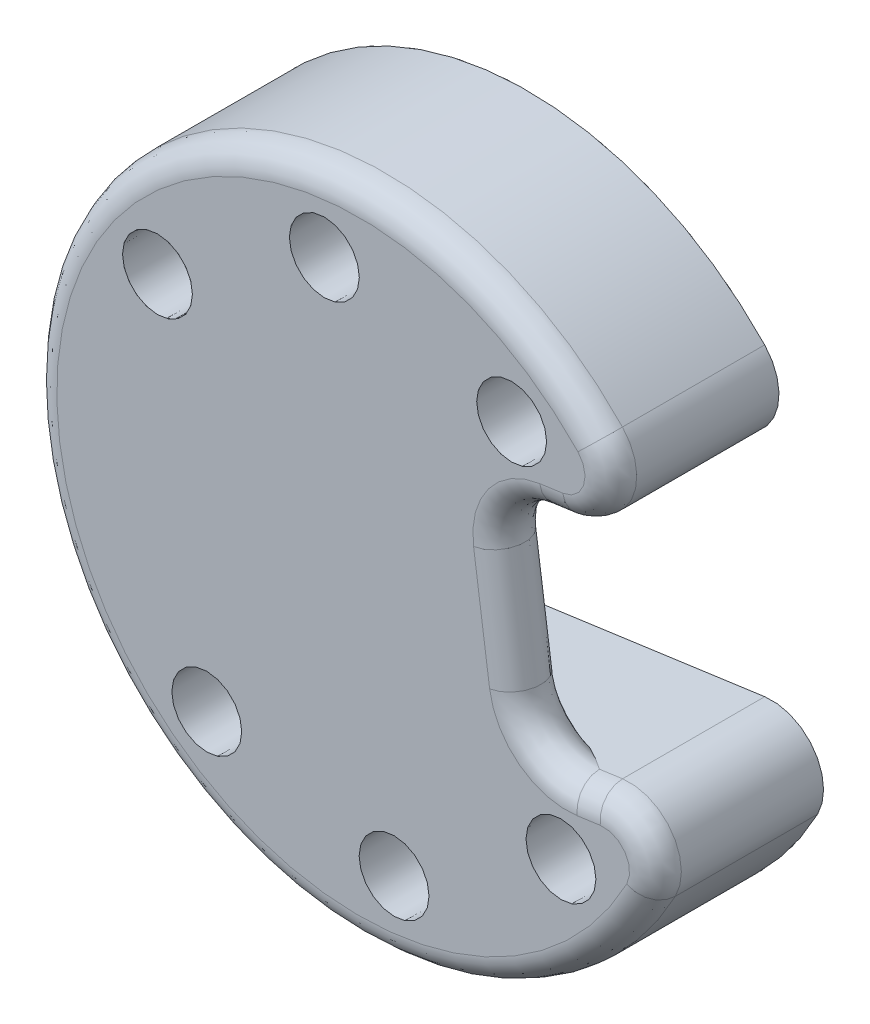
# Autodesk Inventor part: Ring pusher mount
Saved by Autodesk Inventor 2021 (Build 250183000, 183)
## iProperties
Created: 2021-03-14
Part Number: Ring pusher mount
Material: Generic
Document SubType Name: Modeling
Designer: deli
Density: 1 g/cm^3
Appearance: Default
Author: deli
Autodesk Inventor part; units mm, degrees
ref_plane "YZ Plane" through (0, 0, 0) normal (1, 0, 0) x (0, 1, 0)
ref_plane "XZ Plane" through (0, 0, 0) normal (0, 1, 0) x (-1, 0, 0)
ref_plane "XY Plane" through (0, 0, 0) normal (0, 0, 1) x (1, 0, 0)
sketch "Sketch1" plane through (0, 0, 0) normal (0, 0, 1) x (1, 0, 0)
  circle A0 centre (-27.5687, -14.0464) radius 12.6962 projected
  circle A1 centre (-27.5687, -14.0464) radius 3.81 projected
  circle A2 centre (-26.22, -23.732) radius 1.3525 projected
  circle A3 centre (-33.4637, -21.8488) radius 1.3525 projected
  circle A4 centre (-37.2542, -15.3951) radius 1.3525 projected
  circle A5 centre (-35.3711, -8.1514) radius 1.3525 projected
  circle A6 centre (-28.9174, -4.3609) radius 1.3525 projected
  circle A7 centre (-21.6737, -6.244) radius 1.3525 projected
  circle A8 centre (-17.8831, -12.6977) radius 1.3525 projected
  circle A9 centre (-19.7663, -19.9415) radius 1.3525 projected
  line L0 (-9.8275, -15.867) -> (-47.2954, -21.0844)
  line L1 (-47.2954, -21.0844) -> (-48.4677, -12.6656)
  line L2 (-48.4677, -12.6656) -> (-10.9998, -7.4482)
  line L3 (-10.9998, -7.4482) -> (-9.8275, -15.867)
  point P0 (0, 0)
  point P1 (-40.0042, -11.4871)
  point P2 (-16.3055, -8.187)
  point P3 (-15.1331, -16.6058)
  point P4 (-38.8319, -19.9058)
  dimension "d0" = 8.5
  dimension "d1" = 4.25
  dimension "d2" = 4.25
  constraints: 8 end point, 2 parallel, 1 perpendicular
  measures "d0" distance of L0.end L1.end
  measures "d1" distance from line of A8.centre L0
  measures "d2" distance from line of A4.centre L0
extrude "Extrusion1" add sketch "Sketch1" along normal blind 4.5 contours L2 A0 | A0 L0
sketch "Sketch2" plane through (0, 0, 4.5) normal (0, 0, 1) x (1, 0, 0)
  circle A0 centre (-27.5687, -14.0464) radius 12.6962 projected
  circle A1 centre (-19.7663, -19.9415) radius 1.3525 projected
  circle A2 centre (-17.8831, -12.6977) radius 1.3525 projected
  circle A3 centre (-21.6737, -6.244) radius 1.3525 projected
  circle A4 centre (-28.9174, -4.3609) radius 1.3525 projected
  circle A5 centre (-35.3711, -8.1514) radius 1.3525 projected
  circle A6 centre (-37.2542, -15.3951) radius 1.3525 projected
  circle A7 centre (-33.4637, -21.8488) radius 1.3525 projected
  circle A8 centre (-26.22, -23.732) radius 1.3525 projected
  circle A9 centre (-17.8831, -12.6977) radius 4
  arc A10 (-38.8319, -19.9058) -> (-15.1331, -16.6058) centre (-27.5687, -14.0464) ccw projected
  line L0 (-15.1331, -16.6058) -> (-38.8319, -19.9058) projected
  circle A11 centre (-26.22, -23.732) radius 1.3525 projected
  circle A12 centre (-33.4637, -21.8488) radius 1.3525 projected
  circle A13 centre (-19.7663, -19.9415) radius 1.3525 projected
  arc A14 (-16.3055, -8.187) -> (-40.0042, -11.4871) centre (-27.5687, -14.0464) ccw projected
  line L1 (-40.0042, -11.4871) -> (-16.3055, -8.187) projected
  circle A15 centre (-35.3711, -8.1514) radius 1.3525 projected
  circle A16 centre (-28.9174, -4.3609) radius 1.3525 projected
  circle A17 centre (-21.6737, -6.244) radius 1.3525 projected
  line L2 (-15.1331, -16.6058) -> (-38.8319, -19.9058) projected
  line L3 (-21.2588, -17.4588) -> (-22.4311, -9.04)
  line L4 (-40.0042, -11.4871) -> (-16.3055, -8.187) projected
  line L5 (-15.1331, -16.6058) -> (-38.8319, -19.9058) projected
  point P0 (0, 0)
  point P1 (-15.1331, -16.6058)
  point P2 (-16.3055, -8.187)
  dimension "d5" = 8
  constraints: 2 end point, 2 point on line, 1 centre point, 1 coincident, 1 perpendicular, 1 tangent
  measures "d5" diameter of A9
extrude "Extrusion2" add sketch "Sketch2" along normal blind 2 contours L1 A0 | L1 L3 L0 A0 | L0 A0 | A6
fillet "Fillet1" radius 2 5 edges at (-22.4311, -9.04, 5.5) (-21.2588, -17.4588, 5.5) (-15.1331, -16.6058, 5.5) (-15.1331, -16.6058, 2.25) (-16.3055, -8.187, 3.25)
fillet "Fillet2" radius 1 8 edges at (-16.4721, -17.8909, 6.5) (-18.8316, -17.1208, 6.5) (-20.7594, -16.7978, 6.5) (-21.8449, -13.2494, 6.5) (-21.7701, -9.5394, 6.5) (-20.0039, -8.702, 6.5) (-17.9446, -7.3165, 6.5) (-40.1435, -15.7975, 6.5)
fillet "Fillet3" radius 1 3 edges at (-21.7701, -9.5394, 4.5) (-20.7594, -16.7978, 4.5) (-21.8449, -13.2494, 4.5)
equation "\"d2\" = d1"
body "Solid1"
